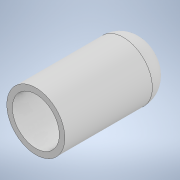
# Autodesk Inventor part: FDMSiCPrintHead_V3
Saved by Autodesk Inventor 2021 (Build 250183000, 183)
## iProperties
Created: 2021-12-13
Part Number: FDMSiCPrintHead_V3
Material: Generic
Document SubType Name: Sheet Metal
Designer: Unit-005
Density: 1 g/cm^3
Sheet Metal Rule: Default
Appearance: Default
Author: Unit-005
## iProperties of the stored document _3DPrint.ipt
Created: 2021-12-13
Part Number: _3DPrint
Material: Generic
Document SubType Name: Modeling
Designer: Unit-005
Density: 1 g/cm^3
Appearance: Default
Author: Unit-005
Autodesk Inventor part; units mm, degrees
ref_plane "YZ Plane" through (0, 0, 0) normal (1, 0, 0) x (0, 1, 0)
ref_plane "XZ Plane" through (0, 0, 0) normal (0, 1, 0) x (-1, 0, 0)
ref_plane "XY Plane" through (0, 0, 0) normal (0, 0, 1) x (1, 0, 0)
sketch "Sketch2" plane through (0, 0, 0) normal (0, 0, 1) x (1, 0, 0)
  circle A0 centre (0, 0) radius 22.25
  dimension "d2" = 44.5
  constraints: 1 centre point, 1 coincident
  measures "d2" diameter of A0
extrude "Extrusion1" add sketch "Sketch2" along normal blind 83
sketch "Sketch9" plane through (0, 0, 83) normal (0, 0, 1) x (1, 0, 0)
  circle A0 centre (0, 0) radius 22.25 projected
  line L0 (-31.15, 0) -> (31.15, 0) projected
  line L1 (0, -31.15) -> (0, 31.15) projected
  circle A1 centre (0, 0) radius 18
  dimension "d54" = 36
  constraints: 1 centre point, 1 coincident
  measures "d54" diameter of A1
extrude "Extrusion7" cut sketch "Sketch9" against normal blind 81 contours A1 L1 L0 | L0 L1 A1 | L1 L0 A1 | A1 L0 L1
fillet "Fillet12" radius 10 1 edges at (-18, 0, 2)
sketch "Sketch18" plane through (0, 0, 2) normal (0, 0, 1) x (1, 0, 0)
  line L0 (-31.15, 0) -> (31.15, 0) projected
  line L1 (0, -31.15) -> (0, 31.15) projected
  line L2 (1.55, 2.35) -> (-1.55, 2.35)
  line L3 (-1.55, 2.35) -> (-1.55, -2.35)
  line L4 (-1.55, -2.35) -> (1.55, -2.35)
  line L5 (1.55, -2.35) -> (1.55, 2.35)
  line L6 (1.55, 2.35) -> (-1.55, -2.35) construction
  line L7 (-1.55, 2.35) -> (1.55, -2.35) construction
  point P0 (0, 0)
  dimension "d122" = 3.1
  dimension "d123" = 4.7
  constraints: 12 end point, 2 midpoint, 2 parallel, 1 horizontal, 1 perpendicular
  measures "d122" distance of L4.end L3.end
  measures "d123" distance of L3.end L2.end
extrude "Extrusion15" cut sketch "Sketch18" against normal through all
chamfer "Chamfer8" distance 2 angle 45 4 edges at (1.55, 0, 2) (0, 2.35, 2) (0, -2.35, 2) (-1.55, 0, 2)
fillet "Fillet13" radius 16 1 edges at (-22.25, 0, 0)
equation "\"BendRadius\" = Thickness"
equation "\"BendReliefWidth\" = Thickness"
equation "\"BendReliefDepth\" = 0.5 * Thickness"
equation "\"CornerReliefSize\" = 4 * Thickness"
equation "\"MinimumRemnant\" = 2 * Thickness"
equation "\"TransitionRadius\" = BendRadius"
equation "\"JacobiRadiusSize\" = BendRadius"
equation "\"GapSize\" = Thickness"
equation "\"Thickness\" = 3.048"
body "Solid1"
